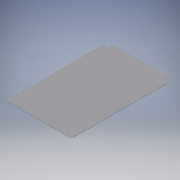
# Autodesk Inventor part: Sheetbottom
Saved by Autodesk Inventor 2016 (Build 200138000, 138)
## iProperties
Created: 2018-11-08
Part Number: Sheetbottom
Material: Generic
Document SubType Name: Sheet Metal
Designer: hovm
Density: 1 g/cm^3
Sheet Metal Rule: Default_mm
Appearance: Default
Author: hovm
Autodesk Inventor part; units mm, degrees
ref_plane "YZ Plane" through (0, 0, 0) normal (1, 0, 0) x (0, 1, 0)
ref_plane "XZ Plane" through (0, 0, 0) normal (0, 1, 0) x (-1, 0, 0)
sketch "Sketch1" plane through (0, 0, 0) normal (0, 0, 1) x (1, 0, 0)
  line L0 (285.6615, 135.8847) -> (589.6615, 135.8847)
  line L1 (589.6615, 135.8847) -> (589.6615, -338.1153)
  line L2 (589.6615, -338.1153) -> (285.6615, -338.1153)
  line L3 (285.6615, -338.1153) -> (285.6615, 135.8847)
  line L4 (285.6615, 135.8847) -> (310.6615, 135.8847)
  line L5 (310.6615, 135.8847) -> (310.6615, 110.8847)
  line L6 (310.6615, 110.8847) -> (285.6615, 110.8847)
  line L7 (285.6615, 110.8847) -> (285.6615, 135.8847)
  line L8 (589.6615, 135.8847) -> (564.6615, 135.8847)
  line L9 (564.6615, 135.8847) -> (564.6615, 110.8847)
  line L10 (564.6615, 110.8847) -> (589.6615, 110.8847)
  line L11 (589.6615, 110.8847) -> (589.6615, 135.8847)
  line L12 (592.6615, 138.6726) -> (592.6615, -341.1153)
  line L13 (596.6615, -341.1153) -> (278.6615, -341.1153)
  line L14 (282.6615, -341.1153) -> (282.6615, 138.6726)
  line L15 (282.8736, 138.8847) -> (592.4493, 138.8847)
  dimension "d44" = 25
  dimension "d45" = 25
  dimension "d46" = 25
  dimension "d47" = 25
  dimension "d80" = 3
  dimension "d81" = 3
  dimension "d82" = 3
  dimension "d83" = 3
  constraints: 32 end point, 6 parallel, 5 horizontal, 3 perpendicular, 2 vertical, 8 other
  measures "d44" distance of L5.end L6.end
  measures "d45" distance of L4.end L5.end
  measures "d46" distance of L10.end L9.end
  measures "d47" distance of L9.end L8.end
  measures "d80" distance from line of L12 L1.end
  measures "d81" distance between parallel lines of L2 L13
  measures "d82" distance between parallel lines of L14 L3
  measures "d83" distance between parallel lines of L4 L15
ref_plane "Work Plane1" through (0, 0, 1) normal (0, 0, 1) x (1, 0, 0)
sketch "Sketch2" plane through (0, 0, 1) normal (0, 0, 1) x (1, 0, 0)
  line L0 (-371, 477) -> (-30.2121, 477) projected
  line L1 (-377, 455) -> (-377, 471) projected
  line L2 (-24.2121, 471) -> (-24.2121, 455) projected
  line L3 (-30.2121, 3) -> (-371, 3) projected
  line L4 (-402, 34) -> (-402, 446) projected
  line L5 (-396, 452) -> (-380, 452) projected
  line L6 (-380, 28) -> (-396, 28) projected
  line L7 (0.7879, 446) -> (0.7879, 34) projected
  point P0 (0, 0)
  point P1 (-317, 467)
  point P2 (-84.2121, 467)
  point P3 (-392, 392)
  point P4 (-392, 88)
  point P5 (-392, 240)
  point P6 (-9.2121, 392)
  point P7 (-9.2121, 240)
  point P8 (-9.2121, 88)
  point P9 (-317, 13)
  point P10 (-84.2121, 13)
  point P11 (-402, 240)
  dimension "d27" = 10
  dimension "d28" = 60
  dimension "d29" = 60
  dimension "d30" = 10
  dimension "d31" = 10
  dimension "d32" = 60
  dimension "d33" = 60
  dimension "d34" = 10
  constraints: 6 horizontal alignment, 6 vertical alignment, 1 midpoint
  measures "d27" distance from line of L0 point (-317, 467)
  measures "d28" distance from line of L1 point (-317, 467)
  measures "d29" distance from line of point (-84.212, 467) L2
  measures "d30" distance from line of point (-317, 13) L3
  measures "d31" distance from line of L4 point (-392, 392)
  measures "d32" distance from line of L5 point (-392, 392)
  measures "d33" distance from line of point (-392, 88) L6
  measures "d34" distance from line of L7 point (-9.212, 392)
extrude "Plate2" add sketch "Sketch1" along normal blind 1 contours L0 L9 L10 L1 L2 L3 L6 L5
hole "Hole2" at (-317, 467, 1) at (-84.2121, 467, 1) at (-392, 392, 1) at (-392, 88, 1) at (-392, 240, 1) at (-9.2121, 392, 1) at (-9.2121, 240, 1) at (-9.2121, 88, 1) at (-317, 13, 1) at (-84.2121, 13, 1) direction (0, 0, -1) diameter 4 depth 1 tip angle 118
chamfer "Corner Chamfer1" distance 6 angle 45 6 edges at (285.6615, 110.8847, 0.5) (310.6615, 135.8847, 0.5) (564.6615, 135.8847, 0.5) (589.6615, 110.8847, 0.5) (589.6615, -338.1153, 0.5) (285.6615, -338.1153, 0.5)
sketch "Sketch3" plane through (0, 0, 1) normal (0, 0, 1) x (1, 0, 0)
  line L0 (291.6615, -338.1153) -> (583.6615, -338.1153) projected
  line L1 (589.6615, 104.8847) -> (589.6615, -332.1153) projected
  line L2 (285.6615, -332.1153) -> (285.6615, 104.8847) projected
  line L3 (316.6615, 135.8847) -> (558.6615, 135.8847) projected
  point P0 (0, 0)
  point P1 (529.6615, -328.1153)
  point P2 (345.6615, -328.1153)
  point P3 (579.6615, -268.1153)
  point P4 (579.6615, -113.6153)
  point P5 (579.6615, 65.8847)
  point P6 (529.6615, 125.8847)
  point P7 (345.6615, 125.8847)
  point P8 (295.6615, 65.8847)
  point P9 (295.6615, -113.6153)
  point P10 (295.6615, -268.1153)
  point P11 (589.6615, -113.6153)
  dimension "d63" = 10
  dimension "d64" = 60
  dimension "d65" = 60
  dimension "d66" = 10
  dimension "d67" = 70
  dimension "d68" = 70
  dimension "d69" = 10
  dimension "d70" = 10
  constraints: 6 horizontal alignment, 6 vertical alignment, 1 midpoint
  measures "d63" distance from line of L0 point (529.661, -328.115)
  measures "d64" distance from line of point (529.661, -328.115) L1
  measures "d65" distance from line of L2 point (345.661, -328.115)
  measures "d66" distance from line of L3 point (529.661, 125.885)
  measures "d67" distance from line of L0 point (579.661, -268.115)
  measures "d68" distance from line of L3 point (579.661, 65.885)
  measures "d69" distance from line of point (579.661, 65.885) L1
  measures "d70" distance from line of L2 point (295.661, 65.885)
hole "Hole3" at (529.6615, -328.1153, 1) at (345.6615, -328.1153, 1) at (579.6615, -268.1153, 1) at (579.6615, -113.6153, 1) at (579.6615, 65.8847, 1) at (529.6615, 125.8847, 1) at (345.6615, 125.8847, 1) at (295.6615, 65.8847, 1) at (295.6615, -113.6153, 1) at (295.6615, -268.1153, 1) direction (0, 0, -1) diameter 4 depth 1 tip angle 118
equation "\"d30\" = d27"
equation "\"d54\" = Thickness"
equation "\"d76\" = Thickness"
equation "\"BendRadius\" = Thickness"
equation "\"BendReliefWidth\" = Thickness"
equation "\"BendReliefDepth\" = 0.5 * Thickness"
equation "\"CornerReliefSize\" = 4 * Thickness"
equation "\"MinimumRemnant\" = 2 * Thickness"
equation "\"TransitionRadius\" = BendRadius"
equation "\"JacobiRadiusSize\" = BendRadius"
equation "\"GapSize\" = Thickness"
equation "\"d26\" = BendRadius"
equation "\"d48\" = BendRadius"
equation "\"Thickness\" = 1"
body "Solid2"
